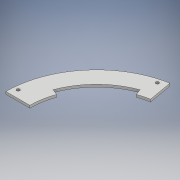
# Autodesk Inventor part: Ring Cover
Saved by Autodesk Inventor 2018 (Build 220112000, 112)
## iProperties
Created: 2018-04-05
Part Number: Ring Cover
Material: Generic
Document SubType Name: Modeling
Designer: anshs
Density: 1 g/cm^3
Appearance: Default
Mass: 2.81216 g
Surface Area: 32.9737 cm^2
Volume: 2.81216 cm^3
Author: anshs
Autodesk Inventor part; units mm, degrees
ref_plane "YZ Plane" through (0, 0, 0) normal (1, 0, 0) x (0, 1, 0)
ref_plane "XZ Plane" through (0, 0, 0) normal (0, 1, 0) x (-1, 0, 0)
ref_plane "XY Plane" through (0, 0, 0) normal (0, 0, 1) x (1, 0, 0)
sketch "Sketch1" plane through (0, 0, 0) normal (0, 0, 1) x (1, 0, 0)
  arc A0 (-12.5027, 70.9062) -> (-72, 0) centre (0, 0) ccw
  line L0 (0, 0) -> (-12.5027, 70.9062) construction
  line L1 (0, 0) -> (-72, 0) construction
  arc A1 (-49.8037, 18.1271) -> (-53, 0) centre (0, 0) ccw
  line L2 (0, 0) -> (-49.8037, 18.1271) construction
  line L3 (0, 0) -> (-53, 0) construction
  arc A2 (-9.2034, 52.1948) -> (-18.1271, 49.8037) centre (0, 0) ccw
  line L4 (0, 0) -> (-18.1271, 49.8037) construction
  line L5 (0, 0) -> (-9.2034, 52.1948) construction
  arc A3 (-19.8372, 54.5022) -> (-54.5022, 19.8372) centre (0, 0) ccw
  line L6 (0, 0) -> (-19.8372, 54.5022) construction
  line L7 (0, 0) -> (-54.5022, 19.8372) construction
  line L8 (-72, 0) -> (-53, 0)
  line L9 (-12.5027, 70.9062) -> (-9.2034, 52.1948)
  line L10 (-49.8037, 18.1271) -> (-54.5022, 19.8372)
  line L11 (-18.1271, 49.8037) -> (-19.8372, 54.5022)
  dimension "d0" = 80
  dimension "d1" = 72
  dimension "d2" = 20
  dimension "d3" = 10
  dimension "d4" = 50
  dimension "d5" = 53
  dimension "d6" = 53
  dimension "d7" = 58
  constraints: 24 end point, 9 point on circle, 4 centre point, 4 coincident, 4 collinear, 2 point on line, 1 horizontal
  measures "d0" angle of L0 L1
  measures "d1" radius of A0
  measures "d2" angle of L2 L3
  measures "d3" angle of L5 L4
  measures "d4" angle of L6 L7
  measures "d5" radius of A1
  measures "d6" radius of A2
  measures "d7" radius of A3
extrude "Extrusion1" add sketch "Sketch1" along normal blind 2
sketch "Sketch2" plane through (0, 0, 2) normal (0, 0, 1) x (1, 0, 0)
  arc A0 (-12.5027, 70.9062) -> (-72, 0) centre (0, 0) ccw projected
  arc A1 (-49.8037, 18.1271) -> (-53, 0) centre (0, 0) ccw projected
  arc A2 (-19.8372, 54.5022) -> (-54.5022, 19.8372) centre (0, 0) ccw projected
  arc A3 (-9.2034, 52.1948) -> (-18.1271, 49.8037) centre (0, 0) ccw projected
  circle A4 centre (-68.2393, 5.9702) radius 1.25
  circle A5 centre (-17.7291, 66.1659) radius 1.25
  line L0 (-72, 0) -> (-53, 0) projected
  line L1 (-49.8037, 18.1271) -> (-54.5022, 19.8372) projected
  line L2 (-19.8372, 54.5022) -> (-18.1271, 49.8037) projected
  line L3 (-9.2034, 52.1948) -> (-12.5027, 70.9062) projected
  line L4 (-68.2393, 5.9702) -> (0, 0) construction
  line L5 (0, 0) -> (-17.7291, 66.1659) construction
  dimension "d10" = 2.5
  dimension "d11" = 2.5
  dimension "d12" = 5
  dimension "d13" = 5
  dimension "d14" = 70
  dimension "d15" = 72
  dimension "d16" = 68.5
  dimension "d17" = 68.5
  constraints: 4 end point, 2 centre point
  measures "d10" diameter of A4
  measures "d11" diameter of A5
  measures "d12" angle of L0 L4
  measures "d13" angle of L3 L5
  measures "d14" angle of L5 L4
  measures "d15" radius of A0
  measures "d16" distance of L4.start L4.end
  measures "d17" distance of L4.end L5.end
extrude "Extrusion2" cut sketch "Sketch2" against normal up to next contours A4 | A5
body "Solid1"
